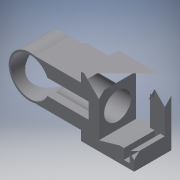
# Autodesk Inventor part: PistonV2
Saved by Autodesk Inventor 2016 (Build 200138000, 138)
## iProperties
Created: 2017-03-04
Part Number: PistonV2
Material: Generic
Document SubType Name: Modeling
Designer: Owner
Density: 1 g/cm^3
Appearance: Default
Author: Owner
Autodesk Inventor part; units mm, degrees
ref_plane "YZ Plane" through (0, 0, 0) normal (1, 0, 0) x (0, 1, 0)
ref_plane "XZ Plane" through (0, 0, 0) normal (0, 1, 0) x (-1, 0, 0)
ref_plane "XY Plane" through (0, 0, 0) normal (0, 0, 1) x (1, 0, 0)
sketch "Sketch1" plane through (0, 0, 0) normal (0, 1, 0) x (-1, 0, 0)
  line L0 (0, 0) -> (7, 0)
  line L1 (7, -23.495) -> (0, -23.495)
  line L2 (-8, -6) -> (-8, 0)
  line L3 (-8, -17.5) -> (-8, -23.5)
  line L4 (-0.01, -3.75) -> (7, -3.75)
  line L5 (-8, -6) -> (-0.01, -3.75)
  line L6 (-8, 0) -> (7, 0)
  line L7 (7, 0) -> (7, -3.75)
  line L8 (-8, -23.5) -> (7, -23.5)
  line L9 (7, -23.5) -> (7, -19.75)
  line L10 (7, -19.75) -> (-0.01, -19.75)
  line L11 (-8, -17.5) -> (-0.01, -19.75)
  line L12 (7, -23.5) -> (0, -23.5)
  line L13 (0, -23.5) -> (0, 0)
  line L14 (0, 0) -> (7, 0)
  line L15 (7, 0) -> (7, -23.5)
  line L16 (-12.74, -21.5) -> (-12.74, -2) projected
  line L17 (-12.74, -2) -> (-10.99, -2) projected
  line L18 (-10.99, -21.5) -> (-10.99, -2) projected
  line L19 (-12.74, -21.5) -> (-10.99, -21.5) projected
  line L20 (-8, -6) -> (-10.99, -6)
  line L21 (-10.99, -6) -> (-10.74, -6)
  line L22 (-10.74, -6) -> (-10.74, -2)
  line L23 (-10.74, -2) -> (-10.74, -1.75)
  line L24 (-10.74, -1.75) -> (-12.74, -1.75)
  line L25 (-12.74, -1.75) -> (-12.99, -1.75)
  line L26 (-12.99, -1.75) -> (-12.99, -6)
  line L27 (-12.99, -6) -> (-14.99, -6)
  line L28 (-14.99, -6) -> (-14.99, 0)
  line L29 (-14.99, 0) -> (-8, 0)
  line L30 (-12.74, -11.75) -> (-14.99, -11.75)
  line L31 (-8, -17.5) -> (-8, -23.5)
  line L32 (-12.74, -2) -> (-12.74, -21.5)
  line L33 (-12.74, -21.5) -> (-10.99, -21.5)
  line L34 (-10.99, -2) -> (-10.99, -21.5)
  line L35 (-8, -17.5) -> (-10.99, -17.5)
  line L36 (-10.99, -17.5) -> (-10.74, -17.5)
  line L37 (-10.74, -17.5) -> (-10.74, -21.5)
  line L38 (-10.74, -21.5) -> (-10.74, -21.75)
  line L39 (-10.74, -21.75) -> (-12.74, -21.75)
  line L40 (-12.74, -21.75) -> (-12.99, -21.75)
  line L41 (-12.99, -21.75) -> (-12.99, -17.5)
  line L42 (-12.99, -17.5) -> (-14.99, -17.5)
  line L43 (-14.99, -17.5) -> (-14.99, -23.5)
  line L44 (-14.99, -23.5) -> (-8, -23.5)
  dimension "d0" = 23.495
  dimension "d1" = 7
  dimension "d8" = 6
  dimension "d10" = 15
  dimension "d11" = 15
  dimension "d51" = 0.25
  dimension "d52" = 0.25
  dimension "d53" = 0.25
  dimension "d54" = 2
  constraints: 76 end point, 16 point on line, 13 symmetric about line, 5 perpendicular, 4 horizontal, 4 parallel, 2 coincident, 1 collinear, 1 midpoint
  measures "d0" distance of L0.start L1.end
  measures "d1" distance of L0.start L0.end
  measures "d8" distance of L11.start L8.start
  measures "d10" distance of L2.end L7.start
  measures "d11" distance of L8.start L8.end
  measures "d51" distance of L20.end L21.end
  measures "d52" distance of L22.end L23.end
  measures "d53" distance of L24.end L25.end
  measures "d54" distance of L26.end L27.end
extrude "Extrusion1" add sketch "Sketch1" along normal blind 14.5 contours L13 L4 L5 L2 L6 | L0 L7 L4 L13 | L2 L20 L22 L23 L24 L25 L26 L27 L28 L29 | L4 L15 L10 L13 | L13 L8 L3 L11 L10 | L10 L9 L1 L13 | L1 L9 L8 L13 | L3 L44 L43 L42 L41 L40 L39 L38 L37 L35
sketch "Sketch2" plane through (-7, 0, -23.5) normal (-1, 0, -0.0000002) x (-0.0000002, 0, 1)
  line L0 (23.5, 0) -> (19.75, 0)
  line L1 (19.75, 0) -> (3.75, 0) projected
  line L2 (19.75, 0) -> (19.75, 14.5) projected
  line L3 (19.75, 0) -> (19.75, 14.5)
  line L4 (6, 0) -> (0, 0) projected
  line L5 (0, 0) -> (3.75, 0)
  line L6 (3.75, 0) -> (3.75, 14.5) projected
  line L7 (3.75, 0) -> (3.75, 14.5)
  line L8 (3.75, 0) -> (19.75, 0)
  line L9 (19.75, 0) -> (19.75, 14.5)
  line L10 (19.75, 14.5) -> (3.75, 14.5)
  line L11 (3.75, 14.5) -> (3.75, 0)
  dimension "d18" = 3.75
  dimension "d19" = 3.75
  constraints: 17 end point, 3 collinear, 2 parallel, 1 horizontal, 1 perpendicular
  measures "d18" distance of L0.start L0.end
  measures "d19" distance of L4.end L1.end
extrude "Extrusion2" add sketch "Sketch2" along normal blind 20
sketch "Sketch3" plane through (0, 0, 0) normal (0, -1, 0) x (1, 0, 0)
  line L0 (-27, -19.75) -> (-27, -3.75) projected
  circle A0 centre (-27, -11.75) radius 8.25
  point P0 (0, 0)
  dimension "d22" = 16.5
  constraints: 1 centre point, 1 midpoint
  measures "d22" diameter of A0
extrude "Extrusion3" add sketch "Sketch3" against normal blind 14.5
sketch "Sketch4" plane through (0, 0, 0) normal (0, -1, 0) x (1, 0, 0)
  arc A0 (-24.9844, -3.75) -> (-24.9844, -19.75) centre (-27, -11.75) ccw projected
  circle A1 centre (-27, -11.75) radius 7.5
  point P0 (0, 0)
  dimension "d25" = 15
  constraints: 1 centre point, 1 coincident
  measures "d25" diameter of A1
extrude "Extrusion4" cut sketch "Sketch4" against normal blind 10.5
sketch "Sketch5" plane through (-27, 10.5, -11.75) normal (0, -1, 0) x (1, 0, 0)
  circle A0 centre (0, 0) radius 7.5 projected
  circle A1 centre (0, 0) radius 7
  point P0 (27, 11.75)
  dimension "d28" = 14
  constraints: 1 centre point, 1 coincident
  measures "d28" diameter of A1
extrude "Extrusion5" cut sketch "Sketch5" against normal blind 10.5 contours A1
sketch "Sketch6" plane through (0, 0, -3.75) normal (1, 0, 0) x (0, 0, -1)
  circle A0 centre (8, 7.25) radius 5.25
  point P0 (-3.75, 0)
  dimension "d31" = 10.5
  constraints: 1 centre point
  measures "d31" diameter of A0
extrude "Extrusion6" cut sketch "Sketch6" against normal blind 30
sketch "Sketch7" plane through (0, 14.5, 0) normal (0, 1, 0) x (1, 0, 0)
  arc A0 (-24.9844, 19.75) -> (-24.9844, 3.75) centre (-27, 11.75) ccw projected
  circle A1 centre (-27, 11.75) radius 8.25
  point P0 (0, 0)
  dimension "d50" = 16.5
  constraints: 1 centre point, 1 coincident
  measures "d50" diameter of A1
extrude "Extrusion7" cut sketch "Sketch7" against normal blind 1
sketch "Sketch9" plane through (0, 0, 0) normal (0, -1, 0) x (1, 0, 0)
  line L0 (-7, -19.75) -> (-24.9844, -19.75) projected
  line L1 (-7, -19.75) -> (-4, -19.75)
  line L2 (-4, -19.75) -> (-4, -16.75)
  line L3 (-7, -3.75) -> (-7, 0) projected
  line L4 (-7, -3.75) -> (-4, -3.75)
  line L5 (-4, -3.75) -> (-4, -6.75)
  line L6 (-4, -16.75) -> (-24, -16.75)
  line L7 (-24, -16.75) -> (-24, -6.75)
  line L8 (-24, -6.75) -> (-4, -6.75)
  line L9 (-4, -6.75) -> (-4, -16.75)
  point P0 (0, 0)
  point P1 (-29.0904, -19.75)
  dimension "d39" = 3
  dimension "d40" = 3
  dimension "d41" = 3
  dimension "d42" = 3
  dimension "d43" = 20
  constraints: 16 end point, 3 horizontal, 2 parallel, 2 perpendicular, 1 vertical
  measures "d39" distance of L0.start L1.end
  measures "d40" distance of L1.end L2.end
  measures "d41" distance of L3.start L4.end
  measures "d42" distance of L4.end L5.end
  measures "d43" distance of L7.end L8.end
extrude "Extrusion9" cut sketch "Sketch9" against normal blind 3
sketch "Sketch10" plane through (0, 3, 0) normal (0, -1, 0) x (1, 0, 0)
  line L0 (-4, -8.6678) -> (-20.1626, -8.6678) projected
  line L1 (-4, -6.75) -> (-4, -8.6678) projected
  line L2 (-21.4098, -6.75) -> (-4, -6.75) projected
  line L3 (-20.1626, -14.8322) -> (-4, -14.8322) projected
  line L4 (-4, -16.75) -> (-21.4098, -16.75) projected
  line L5 (-4, -14.8322) -> (-4, -16.75) projected
  arc A0 (-21.4098, -16.75) -> (-20.1626, -14.8322) centre (-27, -11.75) ccw projected
  arc A1 (-20.1626, -8.6678) -> (-21.4098, -6.75) centre (-27, -11.75) ccw projected
  point P0 (0, 0)
extrude "Extrusion10" add sketch "Sketch10" along normal blind 3
sketch "Sketch12" plane through (14.99, 0, -17.5) normal (1, 0, 0) x (0, 0, -1)
  line L0 (-15.5, 11.975) -> (4, 11.975) projected
  line L1 (-17.5, 14.5) -> (-11.5, 14.5) projected
  line L2 (4, 11.975) -> (-15.5, 11.975)
  line L3 (-15.5, 11.975) -> (-15.5, 14.5)
  line L4 (-15.5, 14.5) -> (4, 14.5)
  line L5 (4, 14.5) -> (4, 11.975)
  line L6 (6, 0) -> (6, 14.5) projected
  line L7 (-17.5, 0) -> (-17.5, 14.5) projected
  line L8 (6, 11.975) -> (-17.5, 11.975)
  line L9 (-17.5, 11.975) -> (-17.5, 14.5)
  line L10 (-17.5, 14.5) -> (6, 14.5)
  line L11 (6, 14.5) -> (6, 11.975)
  constraints: 16 end point, 4 parallel, 2 horizontal, 2 perpendicular, 2 point on line
extrude "Extrusion12" add sketch "Sketch12" against normal blind 6.99
body "Solid1"
